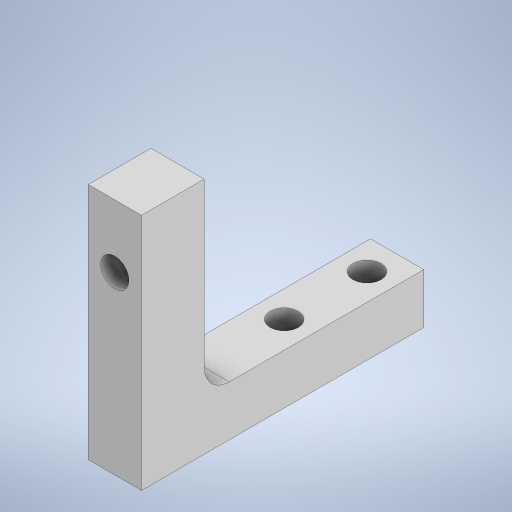
# Autodesk Inventor part: Lconector
Saved by Autodesk Inventor 2024 (Build 280153000, 153)
## iProperties
Created: 2023-12-04
Part Number: Lconector
Material: Generic
Document SubType Name: Modeling
Designer: Nikita
Density: 1 g/cm^3
Appearance: Default
Author: Nikita
Autodesk Inventor part; units mm, degrees
ref_plane "YZ Plane" through (0, 0, 0) normal (1, 0, 0) x (0, 1, 0)
ref_plane "XZ Plane" through (0, 0, 0) normal (0, 1, 0) x (-1, 0, 0)
ref_plane "XY Plane" through (0, 0, 0) normal (0, 0, 1) x (1, 0, 0)
sketch "Sketch1" plane through (0, 0, 0) normal (0, 1, 0) x (-1, 0, 0)
  point P0 (0, 0)
sketch "Sketch2" plane through (0, 0, 0) normal (0, 1, 0) x (-1, 0, 0)
  point P0 (0, 0)
sketch "Sketch3" plane through (0, 0, 0) normal (0, 1, 0) x (-1, 0, 0)
  circle A0 centre (0, 0) radius 2.25
  line L0 (0, 0) -> (0, 27) construction
  line L1 (0, 27) -> (4.25, 27)
  line L2 (4.25, 27) -> (4.25, -18)
  line L3 (4.25, -18) -> (-4.25, -18)
  line L4 (-4.25, -18) -> (-4.25, 27)
  line L5 (-4.25, 27) -> (0, 27)
  dimension "d0" = 4.5
  dimension "d1" = 27
  dimension "d3" = 45
  dimension "d4" = 8.5
  dimension "d5" = 45
  constraints: 12 end point, 3 perpendicular, 1 centre point, 1 coincident, 1 point on line, 1 vertical
  measures "d0" diameter of A0
  measures "d1" distance of L0.start L0.end
  measures "d3" distance of L1.end L2.end
  measures "d4" distance of L2.end L3.end
  measures "d5" distance of L3.end L4.end
extrude "Extrusion1" add sketch "Sketch3" along normal blind 8
sketch "Sketch4" plane through (0, 8, 0) normal (0, 1, 0) x (1, 0, 0)
  line L0 (-4.25, 18) -> (-4.25, -27) projected
  line L1 (-4.25, -27) -> (-4.25, -17)
  line L2 (-4.25, -22) -> (-4.25, -17)
  line L3 (-4.25, -17) -> (4.25, -17)
  line L4 (4.25, -27) -> (4.25, 18) projected
  line L5 (4.25, -27) -> (4.25, -17)
  line L6 (-4.25, -27) -> (4.25, -27)
  point P0 (0, 0)
  dimension "d8" = 10
  constraints: 10 end point, 2 point on line, 1 horizontal
  measures "d8" distance of L0.end L1.end
extrude "Extrusion2" add sketch "Sketch4" along normal blind 30
fillet "Fillet1" radius 4 1 edges at (0, 8, 17)
sketch "Sketch5" plane through (-4.25, 0, 27) normal (0, 0, 1) x (1, 0, 0)
  line L0 (0, 12) -> (0, 38) construction
  line L1 (16.0039, 8) -> (16.0039, 38) construction
  circle A0 centre (4.25, 28) radius 2.25
  line L2 (0, 38) -> (8.5, 38) construction
  line L3 (0, 38) -> (4.25, 38) construction
  line L4 (4.25, 38) -> (4.25, 28) construction
  point P0 (4.25, 0)
  dimension "d12" = 4.5
  dimension "d27" = 4.25
  constraints: 4 end point, 1 centre point, 1 midpoint, 1 perpendicular
  measures "d12" diameter of A0
  measures "d27" distance of L0.end L3.end
extrude "Extrusion3" cut sketch "Sketch5" against normal blind 20
sketch "Sketch7" plane through (0, 8, 0) normal (0, 1, 0) x (1, 0, 0)
  line L0 (0, 0) -> (0, 13.2) construction
  circle A0 centre (0, 13.2) radius 2.25
  dimension "d18" = 13.2
  dimension "d19" = 4.5
  constraints: 2 end point, 1 centre point, 1 coincident, 1 vertical
  measures "d18" distance of L0.start L0.end
  measures "d19" diameter of A0
extrude "Extrusion5" cut sketch "Sketch7" against normal blind 19.4625
body "Solid1"
